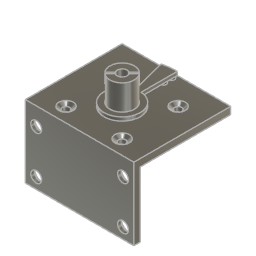
Laser Harp Motor Stand v13 (Autodesk Fusion 360 design; units mm, degrees)
Autodesk Fusion 360 part; units mm, degrees
note: some values were not read from the file. Set by a fixed rule: which sketch regions a step uses.
sketch "Sketch1" plane through (0, 0, 0) normal (0, 0, 1) x (1, 0, 0)
  line L0 (20, -20) -> (-20, -20)
  line L1 (-20, -20) -> (-20, 20)
  line L2 (-20, 20) -> (20, 20)
  line L3 (20, 20) -> (20, -20)
  line L4 (20, -20) -> (-20, 20) construction
  line L5 (-20, -20) -> (20, 20) construction
  line L6 (-20, -20) -> (20, -20)
  line L7 (20, -20) -> (20, 30)
  line L8 (20, 30) -> (-20, 30)
  line L9 (-20, 30) -> (-20, -20)
  circle A0 centre (0, 0) radius 11.25
  circle A1 centre (0, 0) radius 3.5
  line L10 (0, 30) -> (0, -20) construction
  circle A2 centre (0, 27.25) radius 1.75
  circle A3 centre (0, 22.75) radius 1.75
  circle A4 centre (-15.5, 15.5) radius 2
  circle A5 centre (-15.5, -15.5) radius 2
  circle A6 centre (15.5, -15.5) radius 2
  circle A7 centre (15.5, 15.5) radius 2
  line L11 (-20, -20) -> (20, -20)
  line L12 (20, -20) -> (20, -24)
  line L13 (-20, -24) -> (-20, -20)
  line L14 (20, -24) -> (20, -23.5)
  line L15 (20, -23.5) -> (-20, -23.5)
  line L16 (-20, -23.5) -> (-20, -24)
  line L17 (20, 30) -> (30, 30)
  line L18 (30, 30) -> (30, -23.5)
  line L19 (30, -23.5) -> (20, -23.5)
  line L20 (20, -23.5) -> (20, 30)
  line L21 (-20, 30) -> (-30, 30)
  line L22 (-30, 30) -> (-30, -23.5)
  line L23 (-30, -23.5) -> (-20, -23.5)
  line L24 (-20, -23.5) -> (-20, 30)
  line L25 (30, -20) -> (-30, -20)
  point P0 (0, 25.5)
  point P1 (0, 24.5)
  point P2 (0, 29)
  point P3 (0, 21)
  dimension "d1" = 40
  dimension "d2" = 40
  dimension "d3" = 40
  dimension "d4" = 50
  dimension "d5" = 22.5
  dimension "d6" = 7
  dimension "d7" = 3.5
  dimension "d8" = 3.5
  dimension "d9" = 1
  dimension "d10" = 1
  dimension "d11" = 4
  dimension "d12" = 4.5
  dimension "d14" = 360
  dimension "d78" = 3.5
  dimension "d79" = 10
  dimension "d80" = 10
  dimension "d81" = 53.5
  dimension "d82" = 53.5
  dimension "d84" = 3.5
  constraint horizontal L0
  constraint perpendicular L0 L1
  constraint parallel L0 L2
  constraint parallel L1 L3
  constraint coincident L4 A0.centre
  constraint coincident L5 A0.centre
  constraint coincident A0.centre A1.centre
  constraint horizontal L6
  constraint vertical L7
  constraint horizontal L8
  constraint vertical L9
  constraint concentric A0 A1
  constraint midpoint L8 L10.start
  constraint midpoint L0 L10.end
  constraint coincident L10 A2.centre
  constraint coincident L10 A3.centre
  constraint coincident A2 P0
  constraint coincident L10 P0
  constraint coincident A3 P1
  constraint coincident L10 P1
  constraint coincident A2 P2
  constraint coincident L10 P2
  constraint coincident A3 P3
  constraint coincident L10 P3
  constraint coincident L4 A4.centre
  constraint horizontal L11
  constraint vertical L12
  constraint vertical L13
  constraint vertical L14
  constraint horizontal L15
  constraint vertical L16
  constraint horizontal L17
  constraint vertical L18
  constraint horizontal L19
  constraint vertical L20
  constraint horizontal L21
  constraint vertical L22
  constraint horizontal L23
  constraint vertical L24
  constraint coincident L18 L25.start
  constraint coincident L22 L25.end
  constraint perpendicular L22 L25
  measures "d1" distance of L1.end L2.end
  measures "d2" distance of L0.end L1.end
  measures "d3" distance of L0.end L0.start
  measures "d4" distance of L0.end L8.end
  measures "d5" diameter of A0
  measures "d6" diameter of A1
  measures "d7" diameter of A2
  measures "d8" diameter of A3
  measures "d9" distance of P0 P1
  measures "d10" distance of L10.start P2
  measures "d11" diameter of A4
  measures "d12" distance of L2 A4.centre
  measures "d78" distance of L6 L15
  measures "d79" distance of L7.end L17.end
  measures "d80" distance of L8.end L21.end
  measures "d81" distance of L21 L23
  measures "d82" distance of L17 L19
  measures "d84" distance of L23 L25
extrude "Extrude1" add sketch "Sketch1" along normal blind 4 contours L0 L6 L11 L12 L13 L15 L20 L24 L25 | L0 L1 L2 L3 L6 L7 L9 L11 L20 L24 L25 | L12 L18 L19 L20 L25 | L3 L7 L17 L18 L20 L25 | L1 L9 L21 L22 L24 L25 | L13 L22 L23 L24 L25 | L2 L7 L8 L9 L20 L24 makes body 1
extrude "Extrude2" add sketch "Sketch1" along normal blind 2 from surface at 2 contours A0 bodies 1
extrude "Extrude3" add sketch "Sketch1" against normal blind 40 from surface at 4 contours L0 L6 L11 L12 L13 L15 L20 L24 L25 | L12 L18 L19 L20 L25 | L13 L22 L23 L24 L25 bodies 1
sketch "Sketch2" plane through (0, 0, 4) normal (0, 0, 1) x (1, 0, 0)
  circle A0 centre (0, 0) radius 2.75
  circle A1 centre (0, 0) radius 6.75
  circle A2 centre (0, 0) radius 10
  line L0 (0, 0) -> (0, 30) construction
  line L1 (0, 30) -> (0.5, 30)
  line L2 (0.5, 30) -> (0.5, 0)
  line L3 (0.5, 0) -> (0, 0)
  line L4 (0, 0) -> (0, 30)
  line L5 (-0.5, 30) -> (-0.5, 0)
  line L6 (0, 30) -> (-0.5, 30)
  circle A3 centre (0, 0) radius 3.5
  circle A4 centre (0, 22.75) radius 1.75
  circle A5 centre (0, 27.25) radius 1.75
  circle A6 centre (-15.5, 15.5) radius 2
  circle A7 centre (-15.5, -15.5) radius 2
  circle A8 centre (15.5, 15.5) radius 2
  circle A9 centre (15.5, -15.5) radius 2
  line L7 (30, 30) -> (-30, 30)
  line L8 (-30, -23.5) -> (30, -23.5)
  line L9 (30, -23.5) -> (30, 30)
  line L10 (-30, 30) -> (-30, -23.5)
  arc A10 (30, -0.0052) -> (30, 0.0052) centre (0, 0) ccw
  line L11 (0, 0) -> (-7.5149, 29.0435)
  arc A11 (0.5, 29.9958) -> (-7.5149, 29.0435) centre (0, 0) ccw
  arc A12 (-30, 0.0052) -> (-30, -0.0052) centre (0, 0) ccw
  line L12 (0, 0) -> (-0.5, 0)
  line L13 (-2.75, 0) -> (-3.5, 0)
  dimension "d23" = 5.5
  dimension "d24" = 4
  dimension "d31" = 20
  dimension "d52" = 0.5
  constraint coincident A0.centre A1.centre
  constraint concentric A0 A2
  constraint vertical L0
  constraint perpendicular L1 L2
  constraint parallel L1 L3
  constraint parallel L2 L4
  constraint perpendicular L0 L1
  constraint symmetric L0.end L4 L1.start
  constraint symmetric L1.end L4 L5.start
  constraint symmetric L2.end L4 L5.end
  constraint coincident L10 A12.end
  constraint coincident L9 A10.end
  constraint coincident L2 A11.start
  constraint coincident L9 A10.start
  constraint coincident L10 A12.start
  constraint concentric A11 A12
  constraint coincident A3 L13.end
  constraint coincident A0 L13.start
  constraint collinear L12 L13
  measures "d23" diameter of A0
  measures "d31" diameter of A2
  measures "d52" distance of L2 L4
extrude "Extrude4" add sketch "Sketch2" along normal blind 16 separate body contours A0 A3 L11 L13 | A0 L2 A3 L13 | A0 L5 A3 L11 | A1 L2 A3 L11 | A0 L2 L4 A3 | A0 L4 L5 A3 | A1 L5 A3 L11 | A1 L2 L4 A3 | A1 L4 L5 A3 makes body 2
sketch "Sketch3" plane through (0, 0, 20) normal (0, 0, 1) x (-1, 0, 0)
  circle A0 centre (0, 0) radius 3
  circle A1 centre (0, 0) radius 5
  line L0 (0, 0) -> (0, -10) construction
  line L1 (0, 0) -> (-21.2132, -21.2132) construction
  line L2 (0, 0) -> (12.5985, 12.5985) construction
  line L3 (9.2466, 9.2466) -> (-8.7465, -8.7465)
  circle A2 centre (0, 0) radius 3
  circle A3 centre (0, 0) radius 5
  circle A4 centre (0, 0) radius 2.75
  circle A5 centre (0, 0) radius 6.75
  line L4 (5.2382, 5.2382) -> (-5.6662, -5.6662)
  line L5 (-5.6662, -5.6662) -> (-6.0198, -5.3126)
  line L6 (-6.0198, -5.3126) -> (4.8846, 5.5917)
  line L7 (4.8846, 5.5917) -> (5.2382, 5.2382)
  line L8 (-5.3126, -6.0198) -> (5.5917, 4.8846)
  line L9 (5.5917, 4.8846) -> (5.2382, 5.2382)
  line L10 (-5.3126, -6.0198) -> (-5.6662, -5.6662)
  dimension "d57" = 30
  dimension "d58" = 45
  dimension "d68" = 0.5
  constraint coincident A0.centre A1.centre
  constraint vertical L0
  constraint parallel L1 L2
  constraint coincident L1 L3.end
  constraint parallel L1 L3
  constraint perpendicular L4 L5
  constraint parallel L4 L6
  constraint parallel L5 L7
  constraint coincident L1 L4.end
  constraint parallel L1 L4
  constraint symmetric L5.end L4 L8.start
  constraint symmetric L6.end L4 L8.end
  measures "d57" distance of A0.centre L1.end
  measures "d58" angle of L0 L1
  measures "d68" distance of L4.start L6.end
extrude "Extrude8" add sketch "Sketch2" along normal blind 2 separate body contours A1 A2 L5 L11 | A1 A2 L2 L11 | A1 A2 L2 L4 | A1 A2 L4 L5 | A2 L5 A4 A5 L11 A11 | A2 L2 L4 A4 | A2 L4 L5 A4 | L2 L4 A4 | L5 A4 | L4 L5 A4 | L4 L5 A5 A11 | L5 L6 L7 A11 | L2 L4 A4 A5 | L4 L5 A4 A5 | L4 L5 A5 | L5 A5 | L2 L4 A5 A11 | L1 L2 L7 A11 | L2 L4 A5 makes body 3
extrude "Extrude10" cut sketch "Sketch3" against normal blind 5 contours A0 L3 A2 A4 L4 L8 | A0 A1 L3 A2 A3 L4 L8 | A0 A1 L3 A2 A3 L4 L8 | A0 L3 A2 A4 L4 L8 | A0 L3 A2 A4 L4 L6 | A0 A1 L3 A2 A3 L4 L6 | L3 A4 L4 L8 | A1 L3 A3 A5 L4 L8 | A0 A1 L3 A2 A3 L4 L6 | A0 L3 A2 A4 L4 L6 | A1 L3 A3 A5 L4 L8 | A1 L3 A3 A5 L4 L6 | L3 A4 L4 L6 | L3 A5 L4 L8 L9 | A1 L3 A3 A5 L4 L6 | L3 A5 L4 L8 L10 | L3 A5 L4 L6 L7 | L3 A5 L4 L5 L6 bodies 3 2
hole "Hole2" at (0, 6.75, 9.8198) direction (0, -1, 0) diameter 2.93 depth 8 tip angle 118 bodies 2 3
thread "Thread2" "ISO Metric profile 3.5 M3.5x0.6 6H" major diameter 3.5995 minor diameter 2.93 pitch 0.6 angle 60 resizes the face on face at (0.6236, 5.3733, 11.1455) on bodies 2
chamfer "Chamfer1" distance 2 distance2 1.5 4 edges at (13.6353, -14.7768, 4) (-17.3647, -14.7768, 4) (-17.3647, 16.2232, 4) (13.6353, 16.2232, 4) measured on face at (-25.8037, 7.1368, 4) measured on face at (-25.8037, 7.1368, 4) measured on face at (-25.8037, 7.1368, 4) measured on face at (-25.8037, 7.1368, 4) on bodies 1
sketch "Sketch4" plane through (0, -20, 0) normal (0, 1, 0) x (-1, 0, 0)
  line L0 (20, 0) -> (-20, 0)
  line L1 (-20, -36) -> (20, -36)
  circle A0 centre (-24, -6) radius 6
  circle A1 centre (-24, -6) radius 3
  circle A2 centre (24, -6) radius 6
  circle A3 centre (-24, -30) radius 6
  circle A4 centre (24, -30) radius 6
  circle A5 centre (24, -6) radius 3
  circle A6 centre (24, -30) radius 3
  circle A7 centre (-24, -30) radius 3
  line L2 (-20, 0) -> (-20, -36)
  line L3 (20, -36) -> (20, 0)
  dimension "d85" = 6
  dimension "d86" = -3
  dimension "d87" = 6
  dimension "d88" = 6
  dimension "d89" = 6
  dimension "d90" = -3
  dimension "d91" = -3
  dimension "d92" = -3
  constraint tangent L0 A0
  constraint tangent L0 A2
  constraint tangent L1 A3
  constraint tangent L1 A4
  measures "d85" radius of A0
  measures "d87" radius of A2
  measures "d88" radius of A3
  measures "d89" radius of A4
extrude "Extrude11" cut sketch "Sketch4" against normal up to surface (3.5 mm away) contours A1 | A5 | A6 | A7 bodies 1
chamfer "Chamfer2" distance 1.5 angle 45 4 edges at (26.797, -20, -4.9152) (-21.203, -20, -4.9152) (-21.203, -20, -28.9152) (26.797, -20, -28.9152) on bodies 1
combine "Combine3" operation add target body 2 tool bodies 3
named bodies: "Motor Stand", "Mirror Holder"
